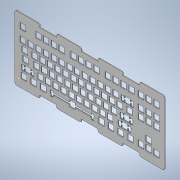
# Autodesk Inventor part: kbplateethan
Saved by Autodesk Inventor 2021 (Build 250183000, 183)
## iProperties
Created: 2023-02-09
Part Number: kbplateethan
Material: Generic
Document SubType Name: Modeling
Designer: ryand
Density: 1 g/cm^3
Appearance: Default
Autodesk Inventor part; units mm, degrees
ref_plane "YZ Plane" through (0, 0, 0) normal (1, 0, 0) x (0, 1, 0)
ref_plane "XZ Plane" through (0, 0, 0) normal (0, 1, 0) x (-1, 0, 0)
ref_plane "XY Plane" through (0, 0, 0) normal (0, 0, 1) x (1, 0, 0)
sketch "Sketch1" plane through (0, 0, 0) normal (0, 0, 1) x (1, 0, 0)
  point P0 (0, 0)
sketch "0" plane through (0, 0, 0) normal (0, 0, 1) x (1, 0, 0)
  line L0 (0, 123.8253) -> (347.6629, 123.8253) construction
  line L1 (347.6629, 123.8253) -> (347.6629, 0) construction
  line L2 (347.6629, 0) -> (0, 0) construction
  line L3 (0, 0) -> (0, 123.8253) construction
  line L4 (123.9669, 16.5254) -> (123.9669, 11.8249)
  line L5 (123.9669, 11.8249) -> (84.343, 11.8249)
  line L6 (84.343, 11.8249) -> (84.343, 15.0551)
  line L7 (84.343, 15.0551) -> (77.5919, 15.0551)
  line L8 (77.5919, 15.0551) -> (77.5919, 11.8249)
  line L9 (77.5919, 11.8249) -> (76.7678, 11.8249)
  line L10 (76.7678, 11.8249) -> (76.7678, 9.0261)
  line L11 (76.7678, 9.0261) -> (77.5919, 9.0261)
  line L12 (77.5919, 9.0261) -> (77.5919, 2.7561)
  line L13 (77.5919, 2.7561) -> (79.3169, 2.7561)
  line L14 (79.3169, 2.7561) -> (79.3169, 1.5558)
  line L15 (79.3169, 1.5558) -> (82.6175, 1.5558)
  line L16 (82.6175, 1.5558) -> (82.6175, 2.7561)
  line L17 (82.6175, 2.7561) -> (84.343, 2.7561)
  line L18 (84.343, 2.7561) -> (84.343, 7.225)
  line L19 (84.343, 7.225) -> (123.9669, 7.225)
  line L20 (123.9669, 7.225) -> (123.9669, 2.5259)
  line L21 (123.9669, 2.5259) -> (137.9679, 2.5259)
  line L22 (137.9679, 2.5259) -> (137.9679, 7.225)
  line L23 (137.9679, 7.225) -> (177.5919, 7.225)
  line L24 (177.5919, 7.225) -> (177.5919, 2.7561)
  line L25 (177.5919, 2.7561) -> (179.3169, 2.7561)
  line L26 (179.3169, 2.7561) -> (179.3169, 1.5558)
  line L27 (179.3169, 1.5558) -> (182.6179, 1.5558)
  line L28 (182.6179, 1.5558) -> (182.6179, 2.7561)
  line L29 (182.6179, 2.7561) -> (184.3429, 2.7561)
  line L30 (184.3429, 2.7561) -> (184.3429, 9.0261)
  line L31 (184.3429, 9.0261) -> (185.1669, 9.0261)
  line L32 (185.1669, 9.0261) -> (185.1669, 11.8249)
  line L33 (185.1669, 11.8249) -> (184.3429, 11.8249)
  line L34 (184.3429, 11.8249) -> (184.3429, 15.0551)
  line L35 (184.3429, 15.0551) -> (177.5919, 15.0551)
  line L36 (177.5919, 15.0551) -> (177.5919, 11.8249)
  line L37 (177.5919, 11.8249) -> (137.9679, 11.8249)
  line L38 (137.9679, 11.8249) -> (137.9679, 16.5254)
  line L39 (137.9679, 16.5254) -> (123.9669, 16.5254)
  line L40 (4.9058, 16.5254) -> (18.9053, 16.5254)
  line L41 (18.9053, 16.5254) -> (18.9053, 2.5259)
  line L42 (18.9053, 2.5259) -> (4.9058, 2.5259)
  line L43 (4.9058, 2.5259) -> (4.9058, 16.5254)
  line L44 (28.7169, 16.5254) -> (42.7177, 16.5254)
  line L45 (42.7177, 16.5254) -> (42.7177, 2.5259)
  line L46 (42.7177, 2.5259) -> (28.7169, 2.5259)
  line L47 (28.7169, 2.5259) -> (28.7169, 16.5254)
  line L48 (52.5309, 16.5254) -> (66.5302, 16.5254)
  line L49 (66.5302, 16.5254) -> (66.5302, 2.5259)
  line L50 (66.5302, 2.5259) -> (52.5309, 2.5259)
  line L51 (52.5309, 2.5259) -> (52.5309, 16.5254)
  line L52 (195.4059, 16.5254) -> (209.4049, 16.5254)
  line L53 (209.4049, 16.5254) -> (209.4049, 2.5259)
  line L54 (209.4049, 2.5259) -> (195.4059, 2.5259)
  line L55 (195.4059, 2.5259) -> (195.4059, 16.5254)
  line L56 (219.2169, 16.5254) -> (233.2179, 16.5254)
  line L57 (233.2179, 16.5254) -> (233.2179, 2.5259)
  line L58 (233.2179, 2.5259) -> (219.2169, 2.5259)
  line L59 (219.2169, 2.5259) -> (219.2169, 16.5254)
  line L60 (243.0309, 16.5254) -> (257.0299, 16.5254)
  line L61 (257.0299, 16.5254) -> (257.0299, 2.5259)
  line L62 (257.0299, 2.5259) -> (243.0309, 2.5259)
  line L63 (243.0309, 2.5259) -> (243.0309, 16.5254)
  line L64 (266.8419, 16.5254) -> (280.8429, 16.5254)
  line L65 (280.8429, 16.5254) -> (280.8429, 2.5259)
  line L66 (280.8429, 2.5259) -> (266.8419, 2.5259)
  line L67 (266.8419, 2.5259) -> (266.8419, 16.5254)
  line L68 (293.0369, 16.5254) -> (307.0369, 16.5254)
  line L69 (307.0369, 16.5254) -> (307.0369, 2.5259)
  line L70 (307.0369, 2.5259) -> (293.0369, 2.5259)
  line L71 (293.0369, 2.5259) -> (293.0369, 16.5254)
  line L72 (312.0869, 16.5254) -> (326.0869, 16.5254)
  line L73 (326.0869, 16.5254) -> (326.0869, 2.5259)
  line L74 (326.0869, 2.5259) -> (312.0869, 2.5259)
  line L75 (312.0869, 2.5259) -> (312.0869, 16.5254)
  line L76 (331.1369, 16.5254) -> (345.1369, 16.5254)
  line L77 (345.1369, 16.5254) -> (345.1369, 2.5259)
  line L78 (345.1369, 2.5259) -> (331.1369, 2.5259)
  line L79 (331.1369, 2.5259) -> (331.1369, 16.5254)
  line L80 (14.4308, 35.5753) -> (14.4308, 30.8749)
  line L81 (14.4308, 30.8749) -> (12.9053, 30.8749)
  line L82 (12.9053, 30.8749) -> (12.9053, 34.1051)
  line L83 (12.9053, 34.1051) -> (6.1557, 34.1051)
  line L84 (6.1557, 34.1051) -> (6.1557, 30.8749)
  line L85 (6.1557, 30.8749) -> (5.3302, 30.8749)
  line L86 (5.3302, 30.8749) -> (5.3302, 28.0761)
  line L87 (5.3302, 28.0761) -> (6.1557, 28.0761)
  line L88 (6.1557, 28.0761) -> (6.1557, 21.8061)
  line L89 (6.1557, 21.8061) -> (7.881, 21.8061)
  line L90 (7.881, 21.8061) -> (7.881, 20.6058)
  line L91 (7.881, 20.6058) -> (11.18, 20.6058)
  line L92 (11.18, 20.6058) -> (11.18, 21.8061)
  line L93 (11.18, 21.8061) -> (12.9053, 21.8061)
  line L94 (12.9053, 21.8061) -> (12.9053, 26.275)
  line L95 (12.9053, 26.275) -> (14.4308, 26.275)
  line L96 (14.4308, 26.275) -> (14.4308, 21.5759)
  line L97 (14.4308, 21.5759) -> (28.4303, 21.5759)
  line L98 (28.4303, 21.5759) -> (28.4303, 26.275)
  line L99 (28.4303, 26.275) -> (29.9558, 26.275)
  line L100 (29.9558, 26.275) -> (29.9558, 21.8061)
  line L101 (29.9558, 21.8061) -> (31.6797, 21.8061)
  line L102 (31.6797, 21.8061) -> (31.6797, 20.6058)
  line L103 (31.6797, 20.6058) -> (34.9801, 20.6058)
  line L104 (34.9801, 20.6058) -> (34.9801, 21.8061)
  line L105 (34.9801, 21.8061) -> (36.7053, 21.8061)
  line L106 (36.7053, 21.8061) -> (36.7053, 28.0761)
  line L107 (36.7053, 28.0761) -> (37.5308, 28.0761)
  line L108 (37.5308, 28.0761) -> (37.5308, 30.8749)
  line L109 (37.5308, 30.8749) -> (36.7053, 30.8749)
  line L110 (36.7053, 30.8749) -> (36.7053, 34.1051)
  line L111 (36.7053, 34.1051) -> (29.9558, 34.1051)
  line L112 (29.9558, 34.1051) -> (29.9558, 30.8749)
  line L113 (29.9558, 30.8749) -> (28.4303, 30.8749)
  line L114 (28.4303, 30.8749) -> (28.4303, 35.5753)
  line L115 (28.4303, 35.5753) -> (14.4308, 35.5753)
  line L116 (252.5549, 35.5753) -> (252.5549, 30.8749)
  line L117 (252.5549, 30.8749) -> (251.0309, 30.8749)
  line L118 (251.0309, 30.8749) -> (251.0309, 34.1051)
  line L119 (251.0309, 34.1051) -> (244.2809, 34.1051)
  line L120 (244.2809, 34.1051) -> (244.2809, 30.8749)
  line L121 (244.2809, 30.8749) -> (243.4549, 30.8749)
  line L122 (243.4549, 30.8749) -> (243.4549, 28.0761)
  line L123 (243.4549, 28.0761) -> (244.2809, 28.0761)
  line L124 (244.2809, 28.0761) -> (244.2809, 21.8061)
  line L125 (244.2809, 21.8061) -> (246.0059, 21.8061)
  line L126 (246.0059, 21.8061) -> (246.0059, 20.6058)
  line L127 (246.0059, 20.6058) -> (249.3049, 20.6058)
  line L128 (249.3049, 20.6058) -> (249.3049, 21.8061)
  line L129 (249.3049, 21.8061) -> (251.0309, 21.8061)
  line L130 (251.0309, 21.8061) -> (251.0309, 26.275)
  line L131 (251.0309, 26.275) -> (252.5549, 26.275)
  line L132 (252.5549, 26.275) -> (252.5549, 21.5759)
  line L133 (252.5549, 21.5759) -> (266.5549, 21.5759)
  line L134 (266.5549, 21.5759) -> (266.5549, 26.275)
  line L135 (266.5549, 26.275) -> (268.0809, 26.275)
  line L136 (268.0809, 26.275) -> (268.0809, 21.8061)
  line L137 (268.0809, 21.8061) -> (269.8059, 21.8061)
  line L138 (269.8059, 21.8061) -> (269.8059, 20.6058)
  line L139 (269.8059, 20.6058) -> (273.1049, 20.6058)
  line L140 (273.1049, 20.6058) -> (273.1049, 21.8061)
  line L141 (273.1049, 21.8061) -> (274.8299, 21.8061)
  line L142 (274.8299, 21.8061) -> (274.8299, 28.0761)
  line L143 (274.8299, 28.0761) -> (275.6559, 28.0761)
  line L144 (275.6559, 28.0761) -> (275.6559, 30.8749)
  line L145 (275.6559, 30.8749) -> (274.8299, 30.8749)
  line L146 (274.8299, 30.8749) -> (274.8299, 34.1051)
  line L147 (274.8299, 34.1051) -> (268.0809, 34.1051)
  line L148 (268.0809, 34.1051) -> (268.0809, 30.8749)
  line L149 (268.0809, 30.8749) -> (266.5549, 30.8749)
  line L150 (266.5549, 30.8749) -> (266.5549, 35.5753)
  line L151 (266.5549, 35.5753) -> (252.5549, 35.5753)
  line L152 (45.3871, 35.5753) -> (59.3864, 35.5753)
  line L153 (59.3864, 35.5753) -> (59.3864, 21.5759)
  line L154 (59.3864, 21.5759) -> (45.3871, 21.5759)
  line L155 (45.3871, 21.5759) -> (45.3871, 35.5753)
  line L156 (64.4371, 35.5753) -> (78.4364, 35.5753)
  line L157 (78.4364, 35.5753) -> (78.4364, 21.5759)
  line L158 (78.4364, 21.5759) -> (64.4371, 21.5759)
  line L159 (64.4371, 21.5759) -> (64.4371, 35.5753)
  line L160 (83.4871, 35.5753) -> (97.4864, 35.5753)
  line L161 (97.4864, 35.5753) -> (97.4864, 21.5759)
  line L162 (97.4864, 21.5759) -> (83.4871, 21.5759)
  line L163 (83.4871, 21.5759) -> (83.4871, 35.5753)
  line L164 (102.5369, 35.5753) -> (116.5369, 35.5753)
  line L165 (116.5369, 35.5753) -> (116.5369, 21.5759)
  line L166 (116.5369, 21.5759) -> (102.5369, 21.5759)
  line L167 (102.5369, 21.5759) -> (102.5369, 35.5753)
  line L168 (121.5869, 35.5753) -> (135.5869, 35.5753)
  line L169 (135.5869, 35.5753) -> (135.5869, 21.5759)
  line L170 (135.5869, 21.5759) -> (121.5869, 21.5759)
  line L171 (121.5869, 21.5759) -> (121.5869, 35.5753)
  line L172 (140.6369, 35.5753) -> (154.6369, 35.5753)
  line L173 (154.6369, 35.5753) -> (154.6369, 21.5759)
  line L174 (154.6369, 21.5759) -> (140.6369, 21.5759)
  line L175 (140.6369, 21.5759) -> (140.6369, 35.5753)
  line L176 (159.6869, 35.5753) -> (173.6869, 35.5753)
  line L177 (173.6869, 35.5753) -> (173.6869, 21.5759)
  line L178 (173.6869, 21.5759) -> (159.6869, 21.5759)
  line L179 (159.6869, 21.5759) -> (159.6869, 35.5753)
  line L180 (178.7369, 35.5753) -> (192.7369, 35.5753)
  line L181 (192.7369, 35.5753) -> (192.7369, 21.5759)
  line L182 (192.7369, 21.5759) -> (178.7369, 21.5759)
  line L183 (178.7369, 21.5759) -> (178.7369, 35.5753)
  line L184 (197.7869, 35.5753) -> (211.7869, 35.5753)
  line L185 (211.7869, 35.5753) -> (211.7869, 21.5759)
  line L186 (211.7869, 21.5759) -> (197.7869, 21.5759)
  line L187 (197.7869, 21.5759) -> (197.7869, 35.5753)
  line L188 (216.8369, 35.5753) -> (230.8369, 35.5753)
  line L189 (230.8369, 35.5753) -> (230.8369, 21.5759)
  line L190 (230.8369, 21.5759) -> (216.8369, 21.5759)
  line L191 (216.8369, 21.5759) -> (216.8369, 35.5753)
  line L192 (312.0869, 35.5753) -> (326.0869, 35.5753)
  line L193 (326.0869, 35.5753) -> (326.0869, 21.5759)
  line L194 (326.0869, 21.5759) -> (312.0869, 21.5759)
  line L195 (312.0869, 21.5759) -> (312.0869, 35.5753)
  line L196 (257.3169, 54.6254) -> (257.3169, 49.9249)
  line L197 (257.3169, 49.9249) -> (255.7929, 49.9249)
  line L198 (255.7929, 49.9249) -> (255.7929, 53.155)
  line L199 (255.7929, 53.155) -> (249.0419, 53.155)
  line L200 (249.0419, 53.155) -> (249.0419, 49.9249)
  line L201 (249.0419, 49.9249) -> (248.2179, 49.9249)
  line L202 (248.2179, 49.9249) -> (248.2179, 47.126)
  line L203 (248.2179, 47.126) -> (249.0419, 47.126)
  line L204 (249.0419, 47.126) -> (249.0419, 40.8561)
  line L205 (249.0419, 40.8561) -> (250.7669, 40.8561)
  line L206 (250.7669, 40.8561) -> (250.7669, 39.6559)
  line L207 (250.7669, 39.6559) -> (254.0659, 39.6559)
  line L208 (254.0659, 39.6559) -> (254.0659, 40.8561)
  line L209 (254.0659, 40.8561) -> (255.7929, 40.8561)
  line L210 (255.7929, 40.8561) -> (255.7929, 45.3251)
  line L211 (255.7929, 45.3251) -> (257.3169, 45.3251)
  line L212 (257.3169, 45.3251) -> (257.3169, 40.6261)
  line L213 (257.3169, 40.6261) -> (271.3179, 40.6261)
  line L214 (271.3179, 40.6261) -> (271.3179, 45.3251)
  line L215 (271.3179, 45.3251) -> (272.8419, 45.3251)
  line L216 (272.8419, 45.3251) -> (272.8419, 40.8561)
  line L217 (272.8419, 40.8561) -> (274.5669, 40.8561)
  line L218 (274.5669, 40.8561) -> (274.5669, 39.6559)
  line L219 (274.5669, 39.6559) -> (277.8679, 39.6559)
  line L220 (277.8679, 39.6559) -> (277.8679, 40.8561)
  line L221 (277.8679, 40.8561) -> (279.5929, 40.8561)
  line L222 (279.5929, 40.8561) -> (279.5929, 47.126)
  line L223 (279.5929, 47.126) -> (280.4169, 47.126)
  line L224 (280.4169, 47.126) -> (280.4169, 49.9249)
  line L225 (280.4169, 49.9249) -> (279.5929, 49.9249)
  line L226 (279.5929, 49.9249) -> (279.5929, 53.155)
  line L227 (279.5929, 53.155) -> (272.8419, 53.155)
  line L228 (272.8419, 53.155) -> (272.8419, 49.9249)
  line L229 (272.8419, 49.9249) -> (271.3179, 49.9249)
  line L230 (271.3179, 49.9249) -> (271.3179, 54.6254)
  line L231 (271.3179, 54.6254) -> (257.3169, 54.6254)
  line L232 (9.6669, 54.6254) -> (23.6678, 54.6254)
  line L233 (23.6678, 54.6254) -> (23.6678, 40.6261)
  line L234 (23.6678, 40.6261) -> (9.6669, 40.6261)
  line L235 (9.6669, 40.6261) -> (9.6669, 54.6254)
  line L236 (35.8621, 54.6254) -> (49.8614, 54.6254)
  line L237 (49.8614, 54.6254) -> (49.8614, 40.6261)
  line L238 (49.8614, 40.6261) -> (35.8621, 40.6261)
  line L239 (35.8621, 40.6261) -> (35.8621, 54.6254)
  line L240 (54.9121, 54.6254) -> (68.9114, 54.6254)
  line L241 (68.9114, 54.6254) -> (68.9114, 40.6261)
  line L242 (68.9114, 40.6261) -> (54.9121, 40.6261)
  line L243 (54.9121, 40.6261) -> (54.9121, 54.6254)
  line L244 (73.9621, 54.6254) -> (87.9614, 54.6254)
  line L245 (87.9614, 54.6254) -> (87.9614, 40.6261)
  line L246 (87.9614, 40.6261) -> (73.9621, 40.6261)
  line L247 (73.9621, 40.6261) -> (73.9621, 54.6254)
  line L248 (93.0121, 54.6254) -> (107.0119, 54.6254)
  line L249 (107.0119, 54.6254) -> (107.0119, 40.6261)
  line L250 (107.0119, 40.6261) -> (93.0121, 40.6261)
  line L251 (93.0121, 40.6261) -> (93.0121, 54.6254)
  line L252 (112.0619, 54.6254) -> (126.0619, 54.6254)
  line L253 (126.0619, 54.6254) -> (126.0619, 40.6261)
  line L254 (126.0619, 40.6261) -> (112.0619, 40.6261)
  line L255 (112.0619, 40.6261) -> (112.0619, 54.6254)
  line L256 (131.1119, 54.6254) -> (145.1119, 54.6254)
  line L257 (145.1119, 54.6254) -> (145.1119, 40.6261)
  line L258 (145.1119, 40.6261) -> (131.1119, 40.6261)
  line L259 (131.1119, 40.6261) -> (131.1119, 54.6254)
  line L260 (150.1619, 54.6254) -> (164.1619, 54.6254)
  line L261 (164.1619, 54.6254) -> (164.1619, 40.6261)
  line L262 (164.1619, 40.6261) -> (150.1619, 40.6261)
  line L263 (150.1619, 40.6261) -> (150.1619, 54.6254)
  line L264 (169.2119, 54.6254) -> (183.2119, 54.6254)
  line L265 (183.2119, 54.6254) -> (183.2119, 40.6261)
  line L266 (183.2119, 40.6261) -> (169.2119, 40.6261)
  line L267 (169.2119, 40.6261) -> (169.2119, 54.6254)
  line L268 (188.2619, 54.6254) -> (202.2619, 54.6254)
  line L269 (202.2619, 54.6254) -> (202.2619, 40.6261)
  line L270 (202.2619, 40.6261) -> (188.2619, 40.6261)
  line L271 (188.2619, 40.6261) -> (188.2619, 54.6254)
  line L272 (207.3119, 54.6254) -> (221.3119, 54.6254)
  line L273 (221.3119, 54.6254) -> (221.3119, 40.6261)
  line L274 (221.3119, 40.6261) -> (207.3119, 40.6261)
  line L275 (207.3119, 40.6261) -> (207.3119, 54.6254)
  line L276 (226.3619, 54.6254) -> (240.3619, 54.6254)
  line L277 (240.3619, 54.6254) -> (240.3619, 40.6261)
  line L278 (240.3619, 40.6261) -> (226.3619, 40.6261)
  line L279 (226.3619, 40.6261) -> (226.3619, 54.6254)
  line L280 (7.2871, 73.6754) -> (21.2866, 73.6754)
  line L281 (21.2866, 73.6754) -> (21.2866, 59.6761)
  line L282 (21.2866, 59.6761) -> (7.2871, 59.6761)
  line L283 (7.2871, 59.6761) -> (7.2871, 73.6754)
  line L284 (31.0996, 73.6754) -> (45.0989, 73.6754)
  line L285 (45.0989, 73.6754) -> (45.0989, 59.6761)
  line L286 (45.0989, 59.6761) -> (31.0996, 59.6761)
  line L287 (31.0996, 59.6761) -> (31.0996, 73.6754)
  line L288 (50.1496, 73.6754) -> (64.1489, 73.6754)
  line L289 (64.1489, 73.6754) -> (64.1489, 59.6761)
  line L290 (64.1489, 59.6761) -> (50.1496, 59.6761)
  line L291 (50.1496, 59.6761) -> (50.1496, 73.6754)
  line L292 (69.1996, 73.6754) -> (83.1989, 73.6754)
  line L293 (83.1989, 73.6754) -> (83.1989, 59.6761)
  line L294 (83.1989, 59.6761) -> (69.1996, 59.6761)
  line L295 (69.1996, 59.6761) -> (69.1996, 73.6754)
  line L296 (88.2496, 73.6754) -> (102.2489, 73.6754)
  line L297 (102.2489, 73.6754) -> (102.2489, 59.6761)
  line L298 (102.2489, 59.6761) -> (88.2496, 59.6761)
  line L299 (88.2496, 59.6761) -> (88.2496, 73.6754)
  line L300 (107.2999, 73.6754) -> (121.2989, 73.6754)
  line L301 (121.2989, 73.6754) -> (121.2989, 59.6761)
  line L302 (121.2989, 59.6761) -> (107.2999, 59.6761)
  line L303 (107.2999, 59.6761) -> (107.2999, 73.6754)
  line L304 (126.3499, 73.6754) -> (140.3489, 73.6754)
  line L305 (140.3489, 73.6754) -> (140.3489, 59.6761)
  line L306 (140.3489, 59.6761) -> (126.3499, 59.6761)
  line L307 (126.3499, 59.6761) -> (126.3499, 73.6754)
  line L308 (145.3999, 73.6754) -> (159.3989, 73.6754)
  line L309 (159.3989, 73.6754) -> (159.3989, 59.6761)
  line L310 (159.3989, 59.6761) -> (145.3999, 59.6761)
  line L311 (145.3999, 59.6761) -> (145.3999, 73.6754)
  line L312 (164.4499, 73.6754) -> (178.4489, 73.6754)
  line L313 (178.4489, 73.6754) -> (178.4489, 59.6761)
  line L314 (178.4489, 59.6761) -> (164.4499, 59.6761)
  line L315 (164.4499, 59.6761) -> (164.4499, 73.6754)
  line L316 (183.4999, 73.6754) -> (197.4989, 73.6754)
  line L317 (197.4989, 73.6754) -> (197.4989, 59.6761)
  line L318 (197.4989, 59.6761) -> (183.4999, 59.6761)
  line L319 (183.4999, 59.6761) -> (183.4999, 73.6754)
  line L320 (202.5499, 73.6754) -> (216.5489, 73.6754)
  line L321 (216.5489, 73.6754) -> (216.5489, 59.6761)
  line L322 (216.5489, 59.6761) -> (202.5499, 59.6761)
  line L323 (202.5499, 59.6761) -> (202.5499, 73.6754)
  line L324 (221.5999, 73.6754) -> (235.5989, 73.6754)
  line L325 (235.5989, 73.6754) -> (235.5989, 59.6761)
  line L326 (235.5989, 59.6761) -> (221.5999, 59.6761)
  line L327 (221.5999, 59.6761) -> (221.5999, 73.6754)
  line L328 (240.6499, 73.6754) -> (254.6489, 73.6754)
  line L329 (254.6489, 73.6754) -> (254.6489, 59.6761)
  line L330 (254.6489, 59.6761) -> (240.6499, 59.6761)
  line L331 (240.6499, 59.6761) -> (240.6499, 73.6754)
  line L332 (264.4619, 73.6754) -> (278.4619, 73.6754)
  line L333 (278.4619, 73.6754) -> (278.4619, 59.6761)
  line L334 (278.4619, 59.6761) -> (264.4619, 59.6761)
  line L335 (264.4619, 59.6761) -> (264.4619, 73.6754)
  line L336 (293.0369, 73.6754) -> (307.0369, 73.6754)
  line L337 (307.0369, 73.6754) -> (307.0369, 59.6761)
  line L338 (307.0369, 59.6761) -> (293.0369, 59.6761)
  line L339 (293.0369, 59.6761) -> (293.0369, 73.6754)
  line L340 (312.0869, 73.6754) -> (326.0869, 73.6754)
  line L341 (326.0869, 73.6754) -> (326.0869, 59.6761)
  line L342 (326.0869, 59.6761) -> (312.0869, 59.6761)
  line L343 (312.0869, 59.6761) -> (312.0869, 73.6754)
  line L344 (331.1369, 73.6754) -> (345.1369, 73.6754)
  line L345 (345.1369, 73.6754) -> (345.1369, 59.6761)
  line L346 (345.1369, 59.6761) -> (331.1369, 59.6761)
  line L347 (331.1369, 59.6761) -> (331.1369, 73.6754)
  line L348 (259.6999, 92.7254) -> (259.6999, 88.0249)
  line L349 (259.6999, 88.0249) -> (258.1739, 88.0249)
  line L350 (258.1739, 88.0249) -> (258.1739, 91.255)
  line L351 (258.1739, 91.255) -> (251.4249, 91.255)
  line L352 (251.4249, 91.255) -> (251.4249, 88.0249)
  line L353 (251.4249, 88.0249) -> (250.5989, 88.0249)
  line L354 (250.5989, 88.0249) -> (250.5989, 85.226)
  line L355 (250.5989, 85.226) -> (251.4249, 85.226)
  line L356 (251.4249, 85.226) -> (251.4249, 78.9561)
  line L357 (251.4249, 78.9561) -> (253.1479, 78.9561)
  line L358 (253.1479, 78.9561) -> (253.1479, 77.7559)
  line L359 (253.1479, 77.7559) -> (256.4489, 77.7559)
  line L360 (256.4489, 77.7559) -> (256.4489, 78.9561)
  line L361 (256.4489, 78.9561) -> (258.1739, 78.9561)
  line L362 (258.1739, 78.9561) -> (258.1739, 83.4251)
  line L363 (258.1739, 83.4251) -> (259.6999, 83.4251)
  line L364 (259.6999, 83.4251) -> (259.6999, 78.7261)
  line L365 (259.6999, 78.7261) -> (273.6989, 78.7261)
  line L366 (273.6989, 78.7261) -> (273.6989, 83.4251)
  line L367 (273.6989, 83.4251) -> (275.2249, 83.4251)
  line L368 (275.2249, 83.4251) -> (275.2249, 78.9561)
  line L369 (275.2249, 78.9561) -> (276.9499, 78.9561)
  line L370 (276.9499, 78.9561) -> (276.9499, 77.7559)
  line L371 (276.9499, 77.7559) -> (280.2489, 77.7559)
  line L372 (280.2489, 77.7559) -> (280.2489, 78.9561)
  line L373 (280.2489, 78.9561) -> (281.9739, 78.9561)
  line L374 (281.9739, 78.9561) -> (281.9739, 85.226)
  line L375 (281.9739, 85.226) -> (282.7999, 85.226)
  line L376 (282.7999, 85.226) -> (282.7999, 88.0249)
  line L377 (282.7999, 88.0249) -> (281.9739, 88.0249)
  line L378 (281.9739, 88.0249) -> (281.9739, 91.255)
  line L379 (281.9739, 91.255) -> (275.2249, 91.255)
  line L380 (275.2249, 91.255) -> (275.2249, 88.0249)
  line L381 (275.2249, 88.0249) -> (273.6989, 88.0249)
  line L382 (273.6989, 88.0249) -> (273.6989, 92.7254)
  line L383 (273.6989, 92.7254) -> (259.6999, 92.7254)
  line L384 (2.5246, 92.7254) -> (16.5241, 92.7254)
  line L385 (16.5241, 92.7254) -> (16.5241, 78.7261)
  line L386 (16.5241, 78.7261) -> (2.5246, 78.7261)
  line L387 (2.5246, 78.7261) -> (2.5246, 92.7254)
  line L388 (21.5746, 92.7254) -> (35.5739, 92.7254)
  line L389 (35.5739, 92.7254) -> (35.5739, 78.7261)
  line L390 (35.5739, 78.7261) -> (21.5746, 78.7261)
  line L391 (21.5746, 78.7261) -> (21.5746, 92.7254)
  line L392 (40.6246, 92.7254) -> (54.6239, 92.7254)
  line L393 (54.6239, 92.7254) -> (54.6239, 78.7261)
  line L394 (54.6239, 78.7261) -> (40.6246, 78.7261)
  line L395 (40.6246, 78.7261) -> (40.6246, 92.7254)
  line L396 (59.6746, 92.7254) -> (73.6739, 92.7254)
  line L397 (73.6739, 92.7254) -> (73.6739, 78.7261)
  line L398 (73.6739, 78.7261) -> (59.6746, 78.7261)
  line L399 (59.6746, 78.7261) -> (59.6746, 92.7254)
  line L400 (78.7246, 92.7254) -> (92.7239, 92.7254)
  line L401 (92.7239, 92.7254) -> (92.7239, 78.7261)
  line L402 (92.7239, 78.7261) -> (78.7246, 78.7261)
  line L403 (78.7246, 78.7261) -> (78.7246, 92.7254)
  line L404 (97.7732, 92.7254) -> (111.7739, 92.7254)
  line L405 (111.7739, 92.7254) -> (111.7739, 78.7261)
  line L406 (111.7739, 78.7261) -> (97.7732, 78.7261)
  line L407 (97.7732, 78.7261) -> (97.7732, 92.7254)
  line L408 (116.8229, 92.7254) -> (130.8239, 92.7254)
  line L409 (130.8239, 92.7254) -> (130.8239, 78.7261)
  line L410 (130.8239, 78.7261) -> (116.8229, 78.7261)
  line L411 (116.8229, 78.7261) -> (116.8229, 92.7254)
  line L412 (135.8749, 92.7254) -> (149.8739, 92.7254)
  line L413 (149.8739, 92.7254) -> (149.8739, 78.7261)
  line L414 (149.8739, 78.7261) -> (135.8749, 78.7261)
  line L415 (135.8749, 78.7261) -> (135.8749, 92.7254)
  line L416 (154.9249, 92.7254) -> (168.9239, 92.7254)
  line L417 (168.9239, 92.7254) -> (168.9239, 78.7261)
  line L418 (168.9239, 78.7261) -> (154.9249, 78.7261)
  line L419 (154.9249, 78.7261) -> (154.9249, 92.7254)
  line L420 (173.9749, 92.7254) -> (187.9739, 92.7254)
  line L421 (187.9739, 92.7254) -> (187.9739, 78.7261)
  line L422 (187.9739, 78.7261) -> (173.9749, 78.7261)
  line L423 (173.9749, 78.7261) -> (173.9749, 92.7254)
  line L424 (193.0249, 92.7254) -> (207.0239, 92.7254)
  line L425 (207.0239, 92.7254) -> (207.0239, 78.7261)
  line L426 (207.0239, 78.7261) -> (193.0249, 78.7261)
  line L427 (193.0249, 78.7261) -> (193.0249, 92.7254)
  line L428 (212.0749, 92.7254) -> (226.0739, 92.7254)
  line L429 (226.0739, 92.7254) -> (226.0739, 78.7261)
  line L430 (226.0739, 78.7261) -> (212.0749, 78.7261)
  line L431 (212.0749, 78.7261) -> (212.0749, 92.7254)
  line L432 (231.1249, 92.7254) -> (245.1239, 92.7254)
  line L433 (245.1239, 92.7254) -> (245.1239, 78.7261)
  line L434 (245.1239, 78.7261) -> (231.1249, 78.7261)
  line L435 (231.1249, 78.7261) -> (231.1249, 92.7254)
  line L436 (293.0369, 92.7254) -> (307.0369, 92.7254)
  line L437 (307.0369, 92.7254) -> (307.0369, 78.7261)
  line L438 (307.0369, 78.7261) -> (293.0369, 78.7261)
  line L439 (293.0369, 78.7261) -> (293.0369, 92.7254)
  line L440 (312.0869, 92.7254) -> (326.0869, 92.7254)
  line L441 (326.0869, 92.7254) -> (326.0869, 78.7261)
  line L442 (326.0869, 78.7261) -> (312.0869, 78.7261)
  line L443 (312.0869, 78.7261) -> (312.0869, 92.7254)
  line L444 (331.1369, 92.7254) -> (345.1369, 92.7254)
  line L445 (345.1369, 92.7254) -> (345.1369, 78.7261)
  line L446 (345.1369, 78.7261) -> (331.1369, 78.7261)
  line L447 (331.1369, 78.7261) -> (331.1369, 92.7254)
  line L448 (2.5246, 121.3003) -> (16.5241, 121.3003)
  line L449 (16.5241, 121.3003) -> (16.5241, 107.3013)
  line L450 (16.5241, 107.3013) -> (2.5246, 107.3013)
  line L451 (2.5246, 107.3013) -> (2.5246, 121.3003)
  line L452 (40.6246, 121.3003) -> (54.6239, 121.3003)
  line L453 (54.6239, 121.3003) -> (54.6239, 107.3013)
  line L454 (54.6239, 107.3013) -> (40.6246, 107.3013)
  line L455 (40.6246, 107.3013) -> (40.6246, 121.3003)
  line L456 (59.6746, 121.3003) -> (73.6739, 121.3003)
  line L457 (73.6739, 121.3003) -> (73.6739, 107.3013)
  line L458 (73.6739, 107.3013) -> (59.6746, 107.3013)
  line L459 (59.6746, 107.3013) -> (59.6746, 121.3003)
  line L460 (78.7246, 121.3003) -> (92.7239, 121.3003)
  line L461 (92.7239, 121.3003) -> (92.7239, 107.3013)
  line L462 (92.7239, 107.3013) -> (78.7246, 107.3013)
  line L463 (78.7246, 107.3013) -> (78.7246, 121.3003)
  line L464 (97.7732, 121.3003) -> (111.7739, 121.3003)
  line L465 (111.7739, 121.3003) -> (111.7739, 107.3013)
  line L466 (111.7739, 107.3013) -> (97.7732, 107.3013)
  line L467 (97.7732, 107.3013) -> (97.7732, 121.3003)
  line L468 (126.3499, 121.3003) -> (140.3489, 121.3003)
  line L469 (140.3489, 121.3003) -> (140.3489, 107.3013)
  line L470 (140.3489, 107.3013) -> (126.3499, 107.3013)
  line L471 (126.3499, 107.3013) -> (126.3499, 121.3003)
  line L472 (145.3999, 121.3003) -> (159.3989, 121.3003)
  line L473 (159.3989, 121.3003) -> (159.3989, 107.3013)
  line L474 (159.3989, 107.3013) -> (145.3999, 107.3013)
  line L475 (145.3999, 107.3013) -> (145.3999, 121.3003)
  line L476 (164.4499, 121.3003) -> (178.4489, 121.3003)
  line L477 (178.4489, 121.3003) -> (178.4489, 107.3013)
  line L478 (178.4489, 107.3013) -> (164.4499, 107.3013)
  line L479 (164.4499, 107.3013) -> (164.4499, 121.3003)
  line L480 (183.4999, 121.3003) -> (197.4989, 121.3003)
  line L481 (197.4989, 121.3003) -> (197.4989, 107.3013)
  line L482 (197.4989, 107.3013) -> (183.4999, 107.3013)
  line L483 (183.4999, 107.3013) -> (183.4999, 121.3003)
  line L484 (212.0749, 121.3003) -> (226.0739, 121.3003)
  line L485 (226.0739, 121.3003) -> (226.0739, 107.3013)
  line L486 (226.0739, 107.3013) -> (212.0749, 107.3013)
  line L487 (212.0749, 107.3013) -> (212.0749, 121.3003)
  line L488 (231.1249, 121.3003) -> (245.1239, 121.3003)
  line L489 (245.1239, 121.3003) -> (245.1239, 107.3013)
  line L490 (245.1239, 107.3013) -> (231.1249, 107.3013)
  line L491 (231.1249, 107.3013) -> (231.1249, 121.3003)
  line L492 (250.1749, 121.3003) -> (264.1739, 121.3003)
  line L493 (264.1739, 121.3003) -> (264.1739, 107.3013)
  line L494 (264.1739, 107.3013) -> (250.1749, 107.3013)
  line L495 (250.1749, 107.3013) -> (250.1749, 121.3003)
  line L496 (269.2249, 121.3003) -> (283.2239, 121.3003)
  line L497 (283.2239, 121.3003) -> (283.2239, 107.3013)
  line L498 (283.2239, 107.3013) -> (269.2249, 107.3013)
  line L499 (269.2249, 107.3013) -> (269.2249, 121.3003)
  line L500 (293.0369, 121.3003) -> (307.0369, 121.3003)
  line L501 (307.0369, 121.3003) -> (307.0369, 107.3013)
  line L502 (307.0369, 107.3013) -> (293.0369, 107.3013)
  line L503 (293.0369, 107.3013) -> (293.0369, 121.3003)
  line L504 (312.0869, 121.3003) -> (326.0869, 121.3003)
  line L505 (326.0869, 121.3003) -> (326.0869, 107.3013)
  line L506 (326.0869, 107.3013) -> (312.0869, 107.3013)
  line L507 (312.0869, 107.3013) -> (312.0869, 121.3003)
  line L508 (331.1369, 121.3003) -> (345.1369, 121.3003)
  line L509 (345.1369, 121.3003) -> (345.1369, 107.3013)
  line L510 (345.1369, 107.3013) -> (331.1369, 107.3013)
  line L511 (331.1369, 107.3013) -> (331.1369, 121.3003)
  line L512 (0, 123.8253) -> (347.6629, 0) construction
  line L513 (347.6629, 123.8253) -> (0, 0) construction
  line L514 (353.6629, 133.8253) -> (296.3858, 133.8253) construction
  line L515 (-10, 129.8253) -> (-10, -6)
  line L516 (357.6629, -6) -> (357.6629, 129.8253)
  line L517 (357.6629, 133.8253) -> (-10, -10) construction
  line L518 (-10, 133.8253) -> (357.6629, -10) construction
  arc A0 (-6, 133.8253) -> (-10, 129.8253) centre (-6, 129.8253) ccw construction
  arc A1 (357.6629, 129.8253) -> (353.6629, 133.8253) centre (353.6629, 129.8253) ccw construction
  arc A2 (-10, -6) -> (-6, -10) centre (-6, -6) ccw construction
  line L519 (-6, 141.3253) -> (47.2772, 141.3253)
  line L520 (51.2772, 137.3253) -> (51.2772, 133.8253)
  line L521 (-10, 126.3253) -> (-10, 133.8253)
  line L522 (-10, 141.3253) -> (51.2772, 126.3253) construction
  line L523 (51.2772, 141.3253) -> (-10, 126.3253) construction
  line L524 (-10, 129.8253) -> (-10, 133.8253) construction
  line L525 (-6, 133.8253) -> (-10, 133.8253) construction
  line L526 (-10, 133.8253) -> (-10, 137.3253)
  line L527 (92.1286, 133.8253) -> (92.1286, 137.3253)
  line L528 (96.1286, 141.3253) -> (149.4057, 141.3253)
  line L529 (153.4057, 137.3253) -> (153.4057, 133.8253)
  line L530 (194.2572, 133.8253) -> (194.2572, 137.3253)
  line L531 (198.2572, 141.3253) -> (251.5343, 141.3253)
  line L532 (255.5343, 137.3253) -> (255.5343, 133.8253)
  line L533 (296.3858, 133.8253) -> (296.3858, 137.3253)
  line L534 (300.3858, 141.3253) -> (353.6629, 141.3253)
  line L535 (357.6629, 137.3253) -> (357.6629, 133.8253)
  line L536 (-10, -2.5) -> (51.2772, -2.5) construction
  line L537 (51.2772, -2.5) -> (51.2772, -10) construction
  line L538 (47.2772, -17.5) -> (-6, -17.5)
  line L539 (-10, -13.5) -> (-10, -10)
  line L540 (-10, -2.5) -> (51.2772, -17.5) construction
  line L541 (51.2772, -2.5) -> (-10, -17.5) construction
  line L542 (-10, -10) -> (-10, -2.5)
  line L543 (51.2772, -10) -> (51.2772, -13.5)
  line L544 (92.1286, -13.5) -> (92.1286, -10)
  line L545 (149.4057, -17.5) -> (96.1286, -17.5)
  line L546 (153.4057, -10) -> (153.4057, -13.5)
  line L547 (194.2572, -13.5) -> (194.2572, -10)
  line L548 (251.5343, -17.5) -> (198.2572, -17.5)
  line L549 (255.5343, -10) -> (255.5343, -13.5)
  line L550 (296.3858, -13.5) -> (296.3858, -10)
  line L551 (353.6629, -17.5) -> (300.3858, -17.5)
  line L552 (357.6629, -10) -> (357.6629, -13.5)
  line L553 (51.2772, -10) -> (92.1286, -10)
  line L554 (153.4057, -10) -> (194.2572, -10)
  line L555 (255.5343, -10) -> (296.3858, -10)
  arc A3 (-10, -13.5) -> (-6, -17.5) centre (-6, -13.5) ccw
  arc A4 (47.2772, -17.5) -> (51.2772, -13.5) centre (47.2772, -13.5) ccw
  arc A5 (92.1286, -13.5) -> (96.1286, -17.5) centre (96.1286, -13.5) ccw
  arc A6 (149.4057, -17.5) -> (153.4057, -13.5) centre (149.4057, -13.5) ccw
  arc A7 (194.2572, -13.5) -> (198.2572, -17.5) centre (198.2572, -13.5) ccw
  arc A8 (251.5343, -17.5) -> (255.5343, -13.5) centre (251.5343, -13.5) ccw
  arc A9 (296.3858, -13.5) -> (300.3858, -17.5) centre (300.3858, -13.5) ccw
  arc A10 (353.6629, -17.5) -> (357.6629, -13.5) centre (353.6629, -13.5) ccw
  line L556 (357.6629, -6) -> (357.6629, -10)
  arc A11 (-6, 141.3253) -> (-10, 137.3253) centre (-6, 137.3253) ccw
  arc A12 (51.2772, 137.3253) -> (47.2772, 141.3253) centre (47.2772, 137.3253) ccw
  line L557 (51.2772, 133.8253) -> (-6, 133.8253) construction
  line L558 (92.1286, 133.8253) -> (51.2772, 133.8253)
  line L559 (153.4057, 133.8253) -> (92.1286, 133.8253) construction
  line L560 (194.2572, 133.8253) -> (153.4057, 133.8253)
  line L561 (255.5343, 133.8253) -> (194.2572, 133.8253) construction
  line L562 (296.3858, 133.8253) -> (255.5343, 133.8253)
  line L563 (357.6629, 133.8253) -> (357.6629, 129.8253)
  arc A13 (96.1286, 141.3253) -> (92.1286, 137.3253) centre (96.1286, 137.3253) ccw
  arc A14 (153.4057, 137.3253) -> (149.4057, 141.3253) centre (149.4057, 137.3253) ccw
  arc A15 (198.2572, 141.3253) -> (194.2572, 137.3253) centre (198.2572, 137.3253) ccw
  arc A16 (255.5343, 137.3253) -> (251.5343, 141.3253) centre (251.5343, 137.3253) ccw
  arc A17 (300.3858, 141.3253) -> (296.3858, 137.3253) centre (300.3858, 137.3253) ccw
  arc A18 (357.6629, 137.3253) -> (353.6629, 141.3253) centre (353.6629, 137.3253) ccw
  point P0 (173.8315, 61.9127)
  point P1 (173.8315, 61.9127)
  point P2 (20.6386, 133.8253)
  point P3 (20.6386, -10)
  point P4 (2.5246, 107.3013)
  point P5 (2.5246, 78.7261)
  point P6 (9.6669, 40.6261)
  point P7 (345.1369, 2.5259)
  point P8 (326.0869, 2.5259)
  point P9 (307.0369, 2.5259)
  point P10 (280.8429, 2.5259)
  point P11 (257.0299, 2.5259)
  point P12 (233.2179, 2.5259)
  point P13 (209.4049, 2.5259)
  point P14 (66.5302, 2.5259)
  point P15 (42.7177, 2.5259)
  point P16 (18.9053, 2.5259)
  point P17 (77.5919, 2.7561)
  dimension "d1" = 123.8253
  dimension "d2" = 347.6629
  dimension "d3" = 367.6629
  dimension "d4" = 143.8253
  dimension "d5" = 4
  dimension "d6" = 61.2771
  dimension "d7" = 15
  dimension "d15" = 61.2771
  dimension "d16" = 15
  dimension "d24" = 4
  dimension "d25" = 4
  dimension "d26" = 4
  dimension "d27" = 4
  constraints: 1128 end point, 52 tangent, 38 point on circle, 29 parallel, 19 centre point, 14 point on line, 13 equal radius, 10 perpendicular, 9 horizontal, 8 collinear, 8 midpoint, 2 vertical, 1 other
  measures "d1" distance of L3.start L3.end
  measures "d2" distance of L2.start L2.end
  measures "d3" distance of L517.end L518.end
  measures "d4" distance of L518.end L517.start
  measures "d5" radius of A0
  measures "d6" distance of L522.end L521.start
  measures "d7" distance of L523.start L522.end
  measures "d15" distance of L540.end L541.end
  measures "d16" distance of L536.end L540.end
  measures "d24" radius of A3
  measures "d25" radius of A5
  measures "d26" radius of A11
  measures "d27" radius of A13
extrude "Extrusion1" add sketch "0" along normal blind 1.5
sketch "Sketch3" plane through (0, 0, 1.5) normal (0, 0, 1) x (1, 0, 0)
  point P0 (0, 0)
equation "\"d6\" = 0.166667 * d3"
equation "\"d15\" = 0.166667 * d3"
body "Solid1"
